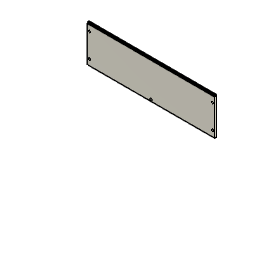
Simple Case V2 - Back (Autodesk Fusion 360 design; units mm, degrees)
Autodesk Fusion 360 part; units mm, degrees
sketch "Sketch1" plane through (0, 72, 0) normal (0, 1, 0) x (-1, 0, 0)
  circle A0 centre (-103, 13) radius 1.425
  circle A1 centre (103, 53) radius 1.425
  circle A2 centre (-103, 53) radius 1.425
  circle A3 centre (103, 13) radius 1.425
  line L0 (-107, 3) -> (107, 3)
  line L1 (107, 3) -> (107, 63)
  line L2 (107, 63) -> (99, 63)
  line L3 (99, 63) -> (99, 5)
  line L4 (-3, 5) -> (-99, 5)
  line L5 (-99, 5) -> (-99, 63)
  line L6 (-99, 63) -> (-107, 63)
  line L7 (-107, 63) -> (-107, 3)
  line L8 (-99, 63) -> (-95.1871, 63)
  line L9 (-95.1871, 63) -> (99, 63)
  line L10 (-106.75, 63) -> (-106.75, 3.25)
  line L11 (-106.75, 3.25) -> (106.75, 3.25)
  line L12 (106.75, 3.25) -> (106.75, 63)
  circle A4 centre (-103, 53) radius 1.75
  circle A5 centre (-103, 13) radius 1.75
  circle A6 centre (103, 13) radius 1.75
  circle A7 centre (103, 53) radius 1.75
  circle A8 centre (0, 6) radius 1.425
  arc A9 (3, 6) -> (-3, 6) centre (0, 6) ccw
  line L13 (-3, 6) -> (-3, 5)
  line L14 (99, 5) -> (3, 5)
  line L15 (3, 5) -> (3, 6)
  circle A10 centre (0, 6) radius 1.75
  dimension "d130" = -0.25
  dimension "d131" = 3.5
  dimension "d132" = 3.5
  dimension "d133" = 3.5
  dimension "d134" = 3.5
  dimension "d148" = 3.5
  constraint coincident L5.end L6.start
  constraint coincident L2.end L3.start
  constraint perpendicular L3 L9
  constraint concentric A2 A4
  constraint concentric A0 A5
  constraint concentric A3 A6
  constraint concentric A1 A7
  constraint concentric A8 A10
  measures "d131" diameter of A4
  measures "d132" diameter of A5
  measures "d133" diameter of A6
  measures "d134" diameter of A7
  measures "d148" diameter of A10
extrude "Extrude1" add sketch "Sketch1" along normal blind 3 contours L2 L3 L4 L5 L6 L10 L11 L12 A9 L13 L14 L15 | L3 L4 L5 L8 L9 A9 L13 L14 L15
sketch "Sketch2" plane through (0, 0, 63) normal (0, 0, 1) x (-1, 0, 0)
  line L0 (106.75, -72) -> (-106.75, -72)
  line L1 (-106.75, -72) -> (-106.75, -75)
  line L2 (-106.75, -75) -> (106.75, -75)
  line L3 (106.75, -75) -> (106.75, -72)
  line L4 (106.75, -73.4) -> (-106.75, -73.4)
  dimension "d137" = 1.6
  constraint coincident L3 L4.start
  constraint coincident L1 L4.end
  constraint perpendicular L1 L4
  measures "d137" distance of L2 L4
extrude "Extrude2" add sketch "Sketch2" along normal blind 2 contours L1 L2 L3 L4
move_body "Move1" bodies 1 to x (1, 0, 0) y (0, 1, 0) z (0, 0, 1) at (0, 130, 0)
